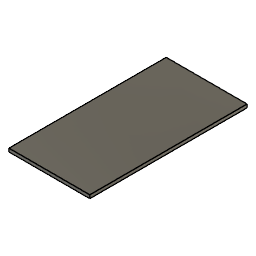
Dak (Autodesk Fusion 360 design; units mm, degrees)
part number: 2026-03-12-09-33-20-472
Autodesk Fusion 360 part; units mm, degrees
sketch "Sketch1" plane through (0, 0, 0) normal (0, 0, 1) x (1, 0, 0)
  line L0 (-33.049, 43.8686) -> (38.951, 43.8686)
  line L1 (38.951, 43.8686) -> (38.951, -96.1314)
  line L2 (38.951, -96.1314) -> (-33.049, -96.1314)
  line L3 (-33.049, -96.1314) -> (-33.049, 43.8686)
  dimension "d1" = 72
  dimension "d2" = 140
  constraint horizontal L0
  constraint vertical L1
  constraint horizontal L2
  constraint vertical L3
  measures "d1" distance of L0.start L0.end
  measures "d2" distance of L0.end L1.end
extrude "Extrude1" add sketch "Sketch1" along normal blind 3
